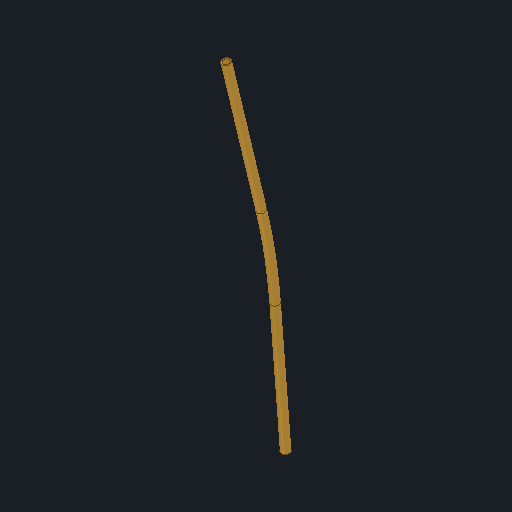
# Autodesk Inventor part: prop_shaft
Saved by Autodesk Inventor 2023 (Build 270158030, 158C)
## iProperties
Created: 2022-04-18
Part Number: prop_shaft
Material: Generic
Document SubType Name: Modeling
Designer: kardo
Density: 1 g/cm^3
Appearance: Brass - Prop shaft
Author: kardo
Autodesk Inventor part; units mm, degrees
ref_plane "YZ Plane" through (0, 0, 0) normal (1, 0, 0) x (0, 1, 0)
ref_plane "XZ Plane" through (0, 0, 0) normal (0, 1, 0) x (-1, 0, 0)
ref_plane "XY Plane" through (0, 0, 0) normal (0, 0, 1) x (1, 0, 0)
derived "stencil_frame.ipt"
sketch "sk_drivetrain_profile" plane through (6, 0, 0) normal (1, 0, 0) x (0, 1, 0)
  line L0 (-529.1844, 0) -> (410.1064, 0) construction
  line L1 (-345, 3089.1136) -> (-345, -1866.0023) construction
  line L2 (0, 3089.1136) -> (0, -1866.0023) construction
  line L3 (-133.5978, 53.515) -> (-127.0613, 26.2887)
  line L4 (-377, 0) -> (-313.1973, 5.0214)
  line L5 (-130.3296, 39.9018) -> (-228.255, 16.392)
  line L6 (-287.0575, 7.0786) -> (-257.2898, 9.4214) construction
  line L7 (-257.2898, 9.4214) -> (-228.255, 16.392) construction
  line L8 (-127.0613, 26.2887) -> (-127.0613, 21.2887) construction
  line L9 (-313.1973, 5.0214) -> (-287.0575, 7.0786)
  line L10 (-844.2225, 3013.4797) -> (331.7536, -1884.8132) construction
  line L11 (-228.9035, 19.0934) -> (-130.9781, 42.6032) construction
  line L12 (-129.681, 37.2005) -> (-227.6064, 13.6907) construction
  line L13 (-228.9035, 19.0934) -> (-227.6064, 13.6907) construction
  spline S0 degree 2 poles (-287.0575, 7.0786) (-257.2898, 9.4214) (-228.255, 16.392) knots 1 1 1 2 2 2
  line L14 (0, 21.3303) -> (-241.5001, 18.9703) construction
  line L15 (-48.9052, 22.0524) -> (-303.0418, 19.569) construction
  point P0 (0, 0)
  point P1 (-216.498, 19.2146)
  point P2 (-204.0926, 19.3359)
  point P3 (-198.8819, 20.5868)
ref_plane "plane_motor_mount" through (0, -120.75, 0) normal (0, 0.9723699, 0.2334454) x (-1, 0, 0)
sketch "sk_prop_shaft_profile" plane through (0, -120.75, 0) normal (0, 0.9723699, 0.2334454) x (-1, 0, 0)
  circle A0 centre (-6, 41.0357) radius 2.7781
  point P0 (0, -28.1885)
  dimension "d1" = 5.5563
  constraints: 1 centre point, 1 coincident
  measures "d1" diameter of A0
derived "parameters_powertrain.ipt"
sweep "Sweep1" add profiles "sk_prop_shaft_profile" path "sk_drivetrain_profile" path curves L5 S0 L9 L4
shell "Shell1" thickness 0.7937 removed faces 2 at (5.8387, -377.04, 0.5088) at (6.7723, -130.6251, 41.1329)
equation "\"d1\" = prop_shaft_sleeve_od"
equation "\"prop_shaft_sleeve_od\" = 5.55625"
body "Solid1"
